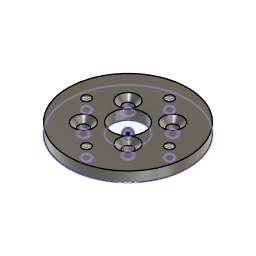
电机固定片-可编辑 (Autodesk Fusion 360 design; units mm, degrees)
Autodesk Fusion 360 part; units mm, degrees
sketch "草图1" plane through (0, 0, 0) normal (0, 0, 1) x (1, 0, 0)
  line L0 (0, 0) -> (51.8, 0) construction
  line L1 (0, 0) -> (0, 48.8683) construction
  circle A0 centre (0, 0) radius 18
  circle A1 centre (0, 0) radius 5
  line L2 (0, 0) -> (20.6611, 20.6611) construction
  line L3 (0, 0) -> (29.2192, 0) construction
  line L4 (0, 0) -> (15.4724, -15.4724) construction
  line L5 (0, 0) -> (21.8812, 0) construction
  point P0 (6.7175, 6.7175)
  point P1 (5.6569, -5.6569)
  point P2 (-6.7175, -6.7175)
  point P3 (-5.6569, 5.6569)
  point P4 (12.5, 0)
  point P5 (-12.5, 0)
  point P6 (0, -12.5)
  point P7 (0, 12.5)
  dimension "d1" = 36
  dimension "d2" = 10
  dimension "d3" = 45
  dimension "d4" = 45
  dimension "d5" = 9.5
  dimension "d6" = 8
  dimension "d7" = 12.5
  constraint coincident L0.start L1.start
  constraint horizontal L0
  constraint perpendicular L0 L1
  constraint concentric A0 A1
  constraint horizontal L3
  constraint horizontal L5
  constraint coincident L2 P0
  constraint coincident L4 P1
  constraint symmetric L4 P0 P2
  constraint symmetric L2 P1 P3
  constraint coincident L3 P4
  constraint symmetric L1 P4 P5
  constraint symmetric L2 P4 P7
  constraint symmetric L2 P5 P6
  measures "d1" diameter of A0
  measures "d2" diameter of A1
  measures "d3" angle of L2 L3
  measures "d4" angle of L4 L5
  measures "d5" distance of L0.start P0
  measures "d6" distance of L0.start P1
  measures "d7" distance of L0.start P4
extrude "拉伸1" add sketch "草图1" along normal blind 3
sketch "草图3" plane through (0, 0, 3) normal (0, 0, 1) x (-1, 0, 0)
  circle A0 centre (0, 0) radius 5
  circle A1 centre (0, 0) radius 18
  line L0 (0, 0) -> (-31, 0) construction
  line L1 (0, 0) -> (17.0073, -17.0073) construction
  line L2 (0, 0) -> (27.2176, 0) construction
  line L3 (0, 0) -> (-13.435, -13.435) construction
  point P0 (-6.7175, -6.7175)
  point P1 (5.6569, -5.6569)
  point P2 (6.7175, 6.7175)
  point P3 (-5.6569, 5.6569)
  dimension "d10" = 45
  dimension "d11" = 45
  dimension "d12" = 9.5
  dimension "d13" = 8
  constraint coincident A0.centre A1.centre
  constraint horizontal L0
  constraint horizontal L2
  constraint midpoint L3 P0
  constraint coincident L1 P1
  constraint symmetric L1 P0 P2
  constraint symmetric L3 P1 P3
  measures "d10" angle of L1 L2
  measures "d11" angle of L0 L3
  measures "d12" distance of A0.centre P0
  measures "d13" distance of A0.centre P1
hole "孔1" at (6.7175, 6.7175, 3) at (-5.6569, 5.6569, 3) at (-6.7175, -6.7175, 3) at (5.6569, -5.6569, 3) direction (0, 0, -1) diameter 3 depth 5 tip angle 118 countersink diameter 6 countersink angle 90
sketch "草图4" plane through (0, 0, 3) normal (0, 0, 1) x (-1, 0, 0)
  circle A0 centre (0, 0) radius 18
  arc A1 (3.5355, -3.5355) -> (-3.5355, 3.5355) centre (0, 0) ccw
  circle A2 centre (5.6569, -5.6569) radius 3
  arc A3 (-3.5355, 3.5355) -> (3.5355, -3.5355) centre (0, 0) ccw
  circle A4 centre (-5.6569, 5.6569) radius 3
  circle A5 centre (-6.7175, -6.7175) radius 3
  circle A6 centre (6.7175, 6.7175) radius 3
  line L0 (0, 0) -> (-28, 0) construction
  line L1 (0, 0) -> (0, -25) construction
  line L2 (0, 0) -> (-17, -17) construction
  point P0 (0, -12.5)
  point P1 (0, 12.5)
  point P2 (-12.5, 0)
  point P3 (12.5, 0)
  dimension "d19" = 12.5
  dimension "d20" = 45
  constraint coincident A0.centre A1.centre
  constraint horizontal L0
  constraint perpendicular L0 L1
  constraint coincident L1 P0
  constraint symmetric L0 P0 P1
  constraint symmetric P0 L2 P2
  constraint symmetric P1 L2 P3
  measures "d19" distance of A0.centre P0
  measures "d20" angle of L0 L2
hole "孔2" at (0, 12.5, 3) at (-12.5, 0, 3) at (0, -12.5, 3) at (12.5, 0, 3) direction (0, 0, -1) diameter 2.529 depth 5 tip angle 118
thread "螺纹1" "ISO Metric profile 3.0 M3x0.5 6H" thread offset 0 thread depth 7.4
sketch "草图5" plane through (0, 0, 0) normal (0, 0, -1) x (1, 0, 0)
  circle A0 centre (0, 12.5) radius 1.2645
  circle A1 centre (0, -12.5) radius 1.2645
  circle A2 centre (-12.5, 0) radius 1.2645
  circle A3 centre (12.5, 0) radius 1.2645
  circle A4 centre (-6.7175, 6.7175) radius 1.5
  circle A5 centre (6.7175, -6.7175) radius 1.5
  circle A6 centre (-5.6569, -5.6569) radius 1.5
  circle A7 centre (5.6569, 5.6569) radius 1.5
  circle A8 centre (0, 0) radius 5
  circle A9 centre (0, 0) radius 18
equation "d7 = ( 25 / 2 ) * 1 mm"
equation "d19 = ( 25 / 2 ) * 1 mm"
